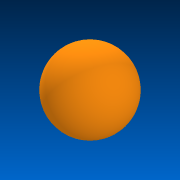
# Autodesk Inventor part: Basketball
Saved by Autodesk Inventor 2022.2 (Build 262287000, 287)
## iProperties
Created: 2022-01-05
Part Number: Basketball
Material: Rubber
Document SubType Name: Modeling
Designer: omard
Density: 0.93 g/cm^3
Appearance: Orange
Mass: 413.233 g
Surface Area: 3498.99 cm^2
Volume: 444.337 cm^3
Author: omard
Autodesk Inventor part; units mm, degrees
ref_plane "YZ Plane" through (0, 0, 0) normal (1, 0, 0) x (0, 1, 0)
ref_plane "XZ Plane" through (0, 0, 0) normal (0, 1, 0) x (-1, 0, 0)
ref_plane "XY Plane" through (0, 0, 0) normal (0, 0, 1) x (1, 0, 0)
sketch "Sketch1" plane through (0, 0, 0) normal (0, 1, 0) x (-1, 0, 0)
  circle A0 centre (0, 0) radius 119.2548
  line L0 (119.2548, 0) -> (-119.2548, 0)
  dimension "d0" = 238.5096
  constraints: 2 coincident, 2 end point, 2 point on circle, 1 centre point, 1 horizontal, 1 midpoint
  measures "d0" diameter of A0
revolve "Revolution1" add sketch "Sketch1" angle 360 about axis through (-119.2548, 0, 0) along (1, 0, 0) picked at (27.435, 51.7312) contours L0 A0
shell "Shell1" thickness 2.54 removed faces 0
body "Solid1"
